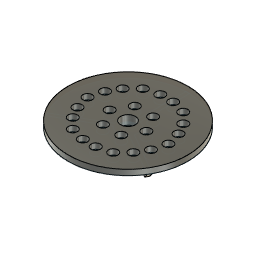
becher halterung v2 (Autodesk Fusion 360 design; units mm, degrees)
Autodesk Fusion 360 part; units mm, degrees
sketch "Skizze1" plane through (0, 0, 0) normal (0, 0, 1) x (1, 0, 0)
  circle A0 centre (0, 0) radius 32.5
  dimension "d1" = 65
  constraint coincident A0.centre origin
  measures "d1" diameter of A0
extrude "Extrusion1" add sketch "Skizze1" along normal blind 3
sketch "Skizze2" plane through (0, 0, 0) normal (0, 0, -1) x (1, 0, 0)
  circle A0 centre (0, 0) radius 32.5
  circle A1 centre (0, 0) radius 5.75
  dimension "d4" = 11.5
  constraint coincident A0.centre A1.centre
  measures "d4" diameter of A1
extrude "Extrusion2" add sketch "Skizze2" along normal blind 4 contours A1
hole "Bohrung1" at (0, 0, 3) direction (0, 0, -1) diameter 4 depth 99 tip angle 118 counterbore diameter 8 counterbore depth 5
sketch "Skizze3" plane through (0, 0, 3) normal (0, 0, 1) x (-1, 0, 0)
  circle A0 centre (0, 0) radius 4
  circle A1 centre (0, 0) radius 32.5
  circle A2 centre (-10, 0.0001) radius 2.5
  circle A3 centre (-22, 0) radius 2.5
  circle A4 centre (-20, 7.5) radius 2.5
  circle A5 centre (-20, -7.5) radius 2.5
  circle A6 centre (-5, -8.6602) radius 2.5
  circle A7 centre (-16.4952, -13.5705) radius 2.5
  circle A8 centre (-11, -19.0526) radius 2.5
  circle A9 centre (-3.5048, -21.0705) radius 2.5
  circle A10 centre (5, -8.6603) radius 2.5
  circle A11 centre (3.5048, -21.0705) radius 2.5
  circle A12 centre (11, -19.0526) radius 2.5
  circle A13 centre (16.4952, -13.5705) radius 2.5
  circle A14 centre (10, -0.0001) radius 2.5
  circle A15 centre (20, -7.5) radius 2.5
  circle A16 centre (22, 0) radius 2.5
  circle A17 centre (20, 7.5) radius 2.5
  circle A18 centre (5, 8.6602) radius 2.5
  circle A19 centre (16.4952, 13.5705) radius 2.5
  circle A20 centre (11, 19.0526) radius 2.5
  circle A21 centre (3.5048, 21.0705) radius 2.5
  circle A22 centre (-5, 8.6603) radius 2.5
  circle A23 centre (-3.5048, 21.0705) radius 2.5
  circle A24 centre (-11, 19.0526) radius 2.5
  circle A25 centre (-16.4952, 13.5705) radius 2.5
  dimension "d12" = 5
  dimension "d13" = 10
  dimension "d14" = 5
  dimension "d15" = 12
  dimension "d18" = 5
  dimension "d19" = 5
  dimension "d21" = 360
  measures "d12" diameter of A2
  measures "d13" distance of A0.centre A2.centre
  measures "d14" diameter of A3
  measures "d15" distance of A2.centre A3.centre
  measures "d18" diameter of A4
extrude "Extrusion3" cut sketch "Skizze3" against normal blind 26 contours A2 | A3 | A4 | A5 | A6 | A7 | A8 | A9 | A10 | A11 | A12 | A13 | A14 | A15 | A16 | A17 | A18 | A19 | A20 | A21 | A22 | A23 | A24 | A25
sketch "Skizze4" plane through (0, 0, 0) normal (0, 0, -1) x (1, 0, 0)
  circle A0 centre (3.5048, -21.0705) radius 2.5
  circle A1 centre (22, 0) radius 2.5
  circle A2 centre (11, 19.0526) radius 2.5
  circle A3 centre (-5, -8.6603) radius 2.5
  circle A4 centre (-22, 0) radius 2.5
  circle A5 centre (-11, 19.0526) radius 2.5
  circle A6 centre (-5, 8.6602) radius 2.5
  circle A7 centre (-10, -0.0001) radius 2.5
  circle A8 centre (5, -8.6602) radius 2.5
  circle A9 centre (16.4952, 13.5705) radius 2.5
  circle A10 centre (20, -7.5) radius 2.5
  circle A11 centre (-3.5048, -21.0705) radius 2.5
  circle A12 centre (11, -19.0526) radius 2.5
  circle A13 centre (20, 7.5) radius 2.5
  circle A14 centre (10, 0.0001) radius 2.5
  circle A15 centre (-11, -19.0526) radius 2.5
  circle A16 centre (-20, 7.5) radius 2.5
  circle A17 centre (-3.5048, 21.0705) radius 2.5
  circle A18 centre (-16.4952, 13.5705) radius 2.5
  circle A19 centre (-16.4952, -13.5705) radius 2.5
  circle A20 centre (-20, -7.5) radius 2.5
  circle A21 centre (3.5048, 21.0705) radius 2.5
  circle A22 centre (16.4952, -13.5705) radius 2.5
  circle A23 centre (5, 8.6603) radius 2.5
  circle A24 centre (0, 0) radius 5.75
  circle A25 centre (0, 0) radius 32.5
  line L0 (1, -32.4807) -> (-1, -32.4807)
  line L1 (-1, -32.4807) -> (-1, -5)
  line L2 (-1, -5) -> (1, -5)
  line L3 (1, -5) -> (1, -32.4807)
  line L4 (28.6291, 15.3743) -> (4.8301, 1.634)
  line L5 (3.8301, 3.366) -> (27.6291, 17.1064)
  line L6 (27.6291, 17.1064) -> (28.6291, 15.3743)
  line L7 (4.8301, 1.634) -> (3.8301, 3.366)
  line L8 (-27.6291, 17.1064) -> (-3.8301, 3.366)
  line L9 (-4.8301, 1.634) -> (-28.6291, 15.3743)
  line L10 (-28.6291, 15.3743) -> (-27.6291, 17.1064)
  line L11 (-3.8301, 3.366) -> (-4.8301, 1.634)
  dimension "d25" = 360
  constraint horizontal L0
  constraint vertical L1
  constraint horizontal L2
  constraint vertical L3
extrude "Extrusion4" add sketch "Skizze4" along normal blind 4 contours A24 L4 L5 L6 | A24 L0 L1 L3 | A24 L8 L9 L10
chamfer "Fase1" distance 4 angle 45 3 edges at (0, 32.4807, -4) (28.1291, -16.2404, -4) (-28.1291, -16.2404, -4)
sketch "Skizze5" plane through (0, 0, 0) normal (0, 0, -1) x (1, 0, 0)
  circle A0 centre (3.5048, -21.0705) radius 2.5
  circle A1 centre (22, 0) radius 2.5
  circle A2 centre (11, 19.0526) radius 2.5
  circle A3 centre (-5, -8.6603) radius 2.5
  circle A4 centre (-22, 0) radius 2.5
  circle A5 centre (-11, 19.0526) radius 2.5
  circle A6 centre (-5, 8.6602) radius 2.5
  circle A7 centre (-10, -0.0001) radius 2.5
  circle A8 centre (5, -8.6602) radius 2.5
  circle A9 centre (16.4952, 13.5705) radius 2.5
  circle A10 centre (20, -7.5) radius 2.5
  circle A11 centre (-3.5048, -21.0705) radius 2.5
  circle A12 centre (11, -19.0526) radius 2.5
  circle A13 centre (20, 7.5) radius 2.5
  circle A14 centre (10, 0.0001) radius 2.5
  circle A15 centre (-11, -19.0526) radius 2.5
  circle A16 centre (-20, 7.5) radius 2.5
  circle A17 centre (-3.5048, 21.0705) radius 2.5
  circle A18 centre (-16.4952, 13.5705) radius 2.5
  circle A19 centre (-16.4952, -13.5705) radius 2.5
  circle A20 centre (-20, -7.5) radius 2.5
  circle A21 centre (3.5048, 21.0705) radius 2.5
  circle A22 centre (16.4952, -13.5705) radius 2.5
  circle A23 centre (5, 8.6603) radius 2.5
  circle A24 centre (0, 0) radius 32.5
  line L0 (-5.4038, 1.9652) -> (-28.6291, 15.3743)
  line L1 (-28.6291, 15.3743) -> (-27.6291, 17.1064)
  line L2 (-27.6291, 17.1064) -> (-4.4038, 3.6972)
  arc A25 (4.4038, 3.6972) -> (-4.4038, 3.6972) centre (0, 0) ccw
  line L3 (4.4038, 3.6972) -> (27.6291, 17.1064)
  line L4 (27.6291, 17.1064) -> (28.6291, 15.3743)
  line L5 (28.6291, 15.3743) -> (5.4038, 1.9652)
  arc A26 (1, -5.6624) -> (5.4038, 1.9652) centre (0, 0) ccw
  line L6 (1, -5.6624) -> (1, -32.4807)
  line L7 (1, -32.4807) -> (-1, -32.4807)
  line L8 (-1, -32.4807) -> (-1, -5.6624)
  arc A27 (-5.4038, 1.9652) -> (-1, -5.6624) centre (0, 0) ccw
